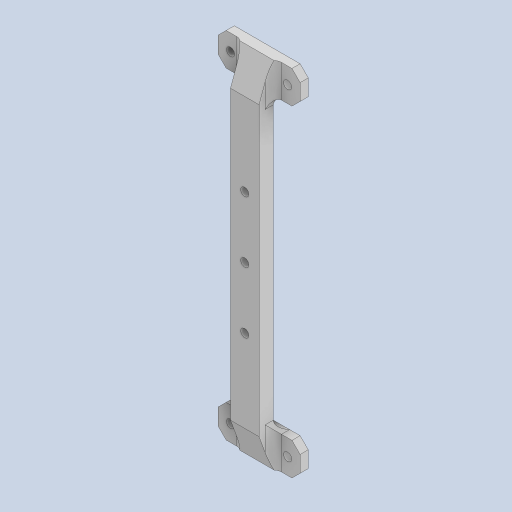
# Autodesk Inventor part: en_shell_1_wid
Saved by Autodesk Inventor 2023 (Build 270158000, 158)
## iProperties
Created: 2021-07-02
Part Number: en_shell_1_wid
Material: Generic
Document SubType Name: Modeling
Designer: Shuang Peng
Density: 1 g/cm^3
Appearance: Default
Author: Shuang Peng
Autodesk Inventor part; units mm, degrees
ref_plane "YZ Plane" through (0, 0, 0) normal (1, 0, 0) x (0, 1, 0)
ref_plane "XZ Plane" through (0, 0, 0) normal (0, 1, 0) x (-1, 0, 0)
ref_plane "XY Plane" through (0, 0, 0) normal (0, 0, 1) x (1, 0, 0)
sketch "Sketch1" plane through (0, 0, 0) normal (0, 0, 1) x (1, 0, 0)
  circle A0 centre (17.0691, -3) radius 1.6 projected
  circle A1 centre (3.0691, -3) radius 1.6 projected
  line L0 (20.1383, 1) -> (0, 1) projected
  line L1 (0, 1) -> (0, -7) projected
  line L2 (0, -7) -> (20.1383, -7) projected
  line L3 (20.1383, 1) -> (20.1383, -7) projected
  circle A2 centre (17.0691, -82) radius 1.6 projected
  circle A3 centre (3.0691, -82) radius 1.6 projected
  line L4 (20.1383, -86) -> (0, -86) projected
  line L5 (20.1383, -86) -> (20.1383, -78) projected
  line L6 (0, -78) -> (20.1383, -78) projected
  line L7 (0, -86) -> (0, -78) projected
  circle A4 centre (3.0691, -3) radius 1
  circle A5 centre (17.0691, -3) radius 1
  circle A6 centre (3.0691, -82) radius 1
  circle A7 centre (17.0691, -82) radius 1
  point P0 (0, 0)
  dimension "d0" = 2
  dimension "d1" = 2
  dimension "d2" = 2
  dimension "d3" = 2
  constraints: 4 centre point, 4 coincident
  measures "d0" diameter of A4
  measures "d1" diameter of A5
  measures "d2" diameter of A6
  measures "d3" diameter of A7
extrude "Extrusion1" add sketch "Sketch1" along normal blind 2 contours A0 | A1 | L3 L2 L1 L0 | A2 | A3 | L4 L7 L6 L5
sketch "Sketch2" plane through (0, 0, 2) normal (0, 0, 1) x (1, 0, 0)
  line L0 (20.1383, -7) -> (20.1383, 1) projected
  line L1 (20.1383, 1) -> (0, 1) projected
  line L2 (0, 1) -> (0, -7) projected
  line L3 (0, -7) -> (20.1383, -7) projected
  circle A0 centre (17.0691, -3) radius 1 projected
  circle A1 centre (3.0691, -3) radius 1 projected
  line L4 (20.1383, -86) -> (20.1383, -78) projected
  line L5 (20.1383, -78) -> (0, -78) projected
  line L6 (0, -78) -> (0, -86) projected
  line L7 (0, -86) -> (20.1383, -86) projected
  circle A2 centre (17.0691, -82) radius 1 projected
  circle A3 centre (3.0691, -82) radius 1 projected
  circle A4 centre (3.0691, -3) radius 1 projected
  line L8 (3.0691, -3) -> (17.0691, -3)
  line L9 (3.0691, -82) -> (17.0691, -82)
  line L10 (10.0691, -82) -> (10.0691, -3)
  line L11 (6.5691, 1) -> (13.5691, 1)
  line L12 (13.5691, 1) -> (13.5691, -86)
  line L13 (13.5691, -86) -> (6.5691, -86)
  line L14 (6.5691, -86) -> (6.5691, 1)
  line L15 (6.5691, 1) -> (13.5691, -86) construction
  line L16 (13.5691, 1) -> (6.5691, -86) construction
  point P0 (0, 0)
  point P1 (10.0691, -42.5)
  dimension "d6" = 7
  dimension "d7" = 87
  constraints: 18 end point, 5 midpoint, 2 horizontal, 2 parallel, 2 perpendicular
  measures "d6" distance of L11.start L11.end
  measures "d7" distance of L11.end L12.end
extrude "Extrusion2" add sketch "Sketch2" along normal blind 3.5 contours L12 L5 L10 L3 | L3 L10 L8 L12 | L12 L8 L14 L1 | L10 L5 L14 L3 | L3 L14 L8 L10 | L12 L9 L10 L5 | L10 L9 L14 L5 | L12 L7 L14 L9
fillet "Fillet1" radius 2 2 edges at (10.0691, -7, 2) (10.0691, -78, 2)
fillet "Fillet2" radius 2 8 edges at (13.5691, -7, 1.0003) (13.5691, -3, 2) (6.5691, -3, 2) (6.5691, -7, 1.0003) (6.5691, -78, 1.0003) (6.5691, -82, 2) (13.5691, -78, 1.0003) (13.5691, -82, 2)
chamfer "Chamfer1" distance 2 angle 45 8 edges at (20.1383, -86, 1) (20.1383, -78, 1) (0, -86, 1) (0, -78, 1) (20.1383, -7, 1) (20.1383, 1, 1) (0, -7, 1) (0, 1, 1)
chamfer "Chamfer2" distance 3 angle 70 1 edges at (10.0691, -86, 5.5) measured on face at (11.6131, -86, 0.7327)
chamfer "Chamfer3" distance 3 angle 70 1 edges at (10.0691, 1, 5.5) measured on face at (11.6131, 1, 0.7327)
sketch "Sketch3" plane through (0, 0, 5.5) normal (0, 0, 1) x (1, 0, 0)
  line L0 (6.5691, -7.2424) -> (13.5691, -7.2424) projected
  line L1 (6.5691, -7.2424) -> (6.5691, -77.7576) projected
  line L2 (13.5691, -77.7576) -> (6.5691, -77.7576) projected
  line L3 (13.5691, -77.7576) -> (13.5691, -7.2424) projected
  line L4 (13.5691, -77.7576) -> (6.5691, -77.7576) projected
  line L5 (10.0691, -77.7576) -> (10.0691, -7.2424)
  circle A0 centre (10.0691, -42.5) radius 1
  line L6 (10.0691, -42.5) -> (10.0691, -27.5)
  circle A1 centre (10.0691, -27.5) radius 1
  line L7 (10.0691, -42.5) -> (10.0691, -57.5)
  circle A2 centre (10.0691, -57.5) radius 1
  point P0 (0, 0)
  dimension "d21" = 2
  dimension "d22" = 15
  dimension "d23" = 2
  dimension "d24" = 15
  dimension "d25" = 2
  constraints: 6 end point, 3 centre point, 3 midpoint, 2 coincident, 2 point on line
  measures "d21" diameter of A0
  measures "d22" distance of L6.start L6.end
  measures "d23" diameter of A1
  measures "d24" distance of L6.start L7.end
  measures "d25" diameter of A2
extrude "Extrusion3" cut sketch "Sketch3" against normal blind 3.5 contours A1 L5 | L5 A1 | A2 L5 | L5 A2 | A0 L5 | L5 A0
body "Solid1"
